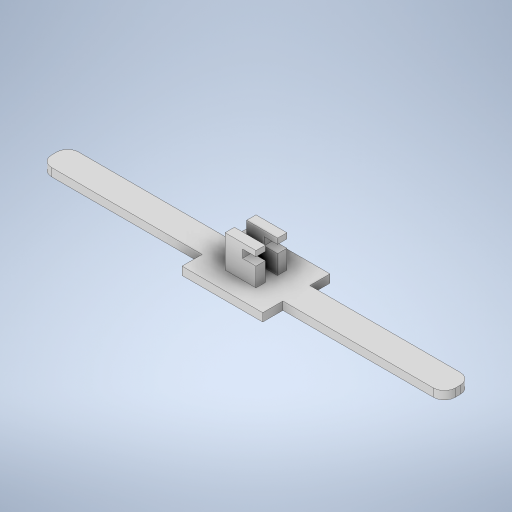
# Autodesk Inventor part: base
Saved by Autodesk Inventor 2024.3 (Build 283343000, 343)
## iProperties
Created: 2024-10-09
Part Number: base
Material: Generic
Document SubType Name: Modeling
Designer: pjcaa
Density: 1 g/cm^3
Appearance: Default
Author: pjcaa
Autodesk Inventor part; units mm, degrees
ref_plane "YZ Plane" through (0, 0, 0) normal (1, 0, 0) x (0, 1, 0)
ref_plane "XZ Plane" through (0, 0, 0) normal (0, 1, 0) x (-1, 0, 0)
ref_plane "XY Plane" through (0, 0, 0) normal (0, 0, 1) x (1, 0, 0)
sketch "Sketch12" plane through (0, 0, 0) normal (0, 0, 1) x (1, 0, 0)
  line L0 (-12.5, 15) -> (12.5, 15)
  line L1 (12.5, 15) -> (12.5, -15)
  line L2 (12.5, -15) -> (-12.5, -15)
  line L3 (-12.5, -15) -> (-12.5, 15)
  line L4 (-12.5, 15) -> (12.5, -15) construction
  line L5 (12.5, 15) -> (-12.5, -15) construction
  point P0 (0, 0)
  dimension "d48" = 25
  dimension "d49" = 30
  constraints: 12 end point, 2 midpoint, 2 parallel, 1 horizontal, 1 perpendicular
  measures "d48" distance of L1.end L2.end
  measures "d49" distance of L0.end L1.end
extrude "Extrusion12" add sketch "Sketch12" along normal blind 3
sketch "Sketch15" plane through (0, 0, 0) normal (0, 0, -1) x (-1, 0, 0)
  line L0 (12.5, -15) -> (-12.5, -15) construction
  line L1 (12.5, 15) -> (12.5, -15) construction
  line L2 (-12.5, 15) -> (12.5, 15) construction
  line L3 (-12.5, -15) -> (-12.5, 15) construction
  line L4 (12.5, 0) -> (-12.5, 0) construction
  line L5 (5, 15) -> (-5, 15)
  line L6 (-5, 15) -> (-5, 75)
  line L7 (-5, 75) -> (5, 75)
  line L8 (5, 75) -> (5, 15)
  line L9 (5, -15) -> (-5, -15)
  line L10 (-5, -15) -> (-5, -75)
  line L11 (-5, -75) -> (5, -75)
  line L12 (5, -75) -> (5, -15)
  point P0 (0, 0)
  point P1 (0, 15)
  point P2 (0, 0)
  dimension "d74" = 10
  dimension "d75" = 60
  constraints: 18 end point, 4 midpoint, 4 symmetric about line, 2 parallel, 1 horizontal, 1 horizontal alignment, 1 perpendicular, 1 vertical alignment
  measures "d74" distance of L6.end L7.end
  measures "d75" distance of L5.end L6.end
extrude "Extrusion15" add sketch "Sketch15" against normal up to surface (3 mm away)
fillet "Fillet1" radius 4 4 edges at (5, 75, 1.5) (-5, 75, 1.5) (-5, -75, 1.5) (5, -75, 1.5)
sketch "Sketch17" plane through (0, 0, 3) normal (0, 0, 1) x (1, 0, 0)
  line L0 (5.75, 5.75) -> (-5.75, 5.75) construction
  line L1 (-5.75, 5.75) -> (-5.75, -5.75) construction
  line L2 (-5.75, -5.75) -> (5.75, -5.75) construction
  line L3 (5.75, -5.75) -> (5.75, 5.75) construction
  line L4 (5.75, 5.75) -> (-5.75, -5.75) construction
  line L5 (-5.75, 5.75) -> (5.75, -5.75) construction
  line L6 (5.75, 5.75) -> (2.25, 5.75)
  line L7 (2.25, 5.75) -> (2.25, -5.75)
  line L8 (2.25, -5.75) -> (5.75, -5.75)
  line L9 (5.75, -5.75) -> (5.75, 5.75)
  line L10 (-5.75, -5.75) -> (-2.25, -5.75)
  line L11 (-2.25, -5.75) -> (-2.25, 5.75)
  line L12 (-2.25, 5.75) -> (-5.75, 5.75)
  line L13 (-5.75, 5.75) -> (-5.75, -5.75)
  point P0 (0, 0)
  dimension "d84" = 11.5
  dimension "d85" = 11.5
  dimension "d86" = 3.5
  dimension "d87" = 3.5
  constraints: 28 end point, 6 parallel, 3 horizontal, 3 perpendicular, 2 midpoint, 2 point on line
  measures "d84" distance of L2.end L1.end
  measures "d85" distance of L0.end L1.end
  measures "d86" distance of L8.end L7.end
  measures "d87" distance of L12.end L11.end
extrude "Extrusion17" add sketch "Sketch17" along normal blind 12
sketch "Sketch18" plane through (-5.75, -5.75, 3) normal (0, -1, 0) x (1, 0, 0)
  line L0 (3.5, 0) -> (0, 0) construction
  line L1 (3.5, 0) -> (3.5, 12) construction
  line L2 (0, 12) -> (3.5, 12) construction
  line L3 (0, 0) -> (0, 12) construction
  line L4 (11.5, 0) -> (8, 0) construction
  line L5 (11.5, 0) -> (11.5, 12) construction
  line L6 (8, 12) -> (11.5, 12) construction
  line L7 (8, 0) -> (8, 12) construction
  line L8 (0, 10) -> (11.5, 10)
  line L9 (11.5, 10) -> (11.5, 7)
  line L10 (11.5, 7) -> (0, 7)
  line L11 (0, 7) -> (0, 10)
  point P0 (5.75, -3)
  dimension "d90" = 2
  dimension "d91" = 3
  constraints: 8 end point, 2 parallel, 2 point on line, 1 horizontal, 1 perpendicular
  measures "d90" distance from line of L8.start L2
  measures "d91" distance between parallel lines of L8 L10
extrude "Extrusion18" cut sketch "Sketch18" against normal blind 5
body "Solid2"
